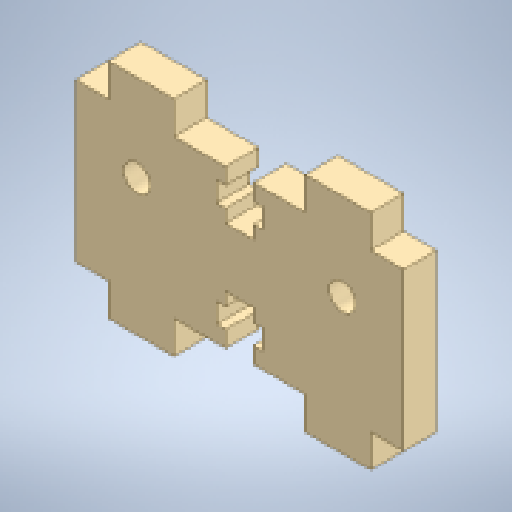
# Autodesk Inventor part: стена_каретки
Saved by Autodesk Inventor 2024 (Build 280153000, 153)
## iProperties
Created: 2026-02-02
Part Number: стена_каретки
Material: Типовые
Document SubType Name: Modeling
Designer: DELL
Density: 1 g/cm^3
Appearance: Пшеничный
Author: DELL
Autodesk Inventor part; units mm, degrees
ref_plane "YZ Plane" through (0, 0, 0) normal (1, 0, 0) x (0, 1, 0)
ref_plane "XZ Plane" through (0, 0, 0) normal (0, 1, 0) x (-1, 0, 0)
ref_plane "XY Plane" through (0, 0, 0) normal (0, 0, 1) x (1, 0, 0)
sketch "Эскиз1" plane through (0, 0, 0) normal (0, 0, 1) x (1, 0, 0)
  line L0 (20, 9.6) -> (-20, 9.6)
  line L1 (-20, 9.6) -> (-20, -9.6)
  line L2 (-20, -9.6) -> (20, -9.6)
  line L3 (20, -9.6) -> (20, 9.6)
  line L4 (20, 9.6) -> (-20, -9.6) construction
  line L5 (-20, 9.6) -> (20, -9.6) construction
  line L6 (-16, 9.6) -> (-8, 9.6)
  line L7 (-8, 9.6) -> (-8, 13.6)
  line L8 (-8, 13.6) -> (-16, 13.6)
  line L9 (-16, 13.6) -> (-16, 9.6)
  line L10 (16, 9.6) -> (8, 9.6)
  line L11 (8, 9.6) -> (8, 13.6)
  line L12 (8, 13.6) -> (16, 13.6)
  line L13 (16, 13.6) -> (16, 9.6)
  line L14 (-16, -9.6) -> (-8, -9.6)
  line L15 (-8, -9.6) -> (-8, -13.6)
  line L16 (-8, -13.6) -> (-16, -13.6)
  line L17 (-16, -13.6) -> (-16, -9.6)
  line L18 (8, -9.6) -> (16, -9.6)
  line L19 (16, -9.6) -> (16, -13.6)
  line L20 (16, -13.6) -> (8, -13.6)
  line L21 (8, -13.6) -> (8, -9.6)
  point P0 (0, 0)
  point P1 (-16, 11.6)
  point P2 (16, -9.6)
  point P3 (8, 9.6)
  point P4 (-8, 9.6)
  dimension "d0" = 40
  dimension "d1" = 19.2
  dimension "d2" = 8
  dimension "d3" = 4
  dimension "d4" = 8
  dimension "d5" = 4
  dimension "d6" = 4
  dimension "d7" = 4
  dimension "d8" = 8
  dimension "d9" = 4
  constraints: 44 end point, 10 parallel, 5 horizontal, 5 perpendicular, 5 point on line, 3 midpoint
  measures "d0" distance of L2.end L1.end
  measures "d1" distance of L1.end L0.end
  measures "d2" distance of L8.end L7.end
  measures "d3" distance of L7.end L6.end
  measures "d4" distance of L11.end L12.end
  measures "d5" distance from line of L1 point (-16, 11.6)
  measures "d6" distance between parallel lines of L13 L3
  measures "d7" distance of L10.end L11.end
  measures "d8" distance of L15.end L16.end
  measures "d9" distance of L14.end L15.end
extrude "Выдавливание1" add sketch "Эскиз1" along normal blind 4
sketch "Эскиз2" plane through (0, 0, 4) normal (0, 0, 1) x (1, 0, 0)
  line L0 (8, 9.6) -> (-8, 9.6) projected
  line L1 (-1.7, 9.6) -> (1.7, 9.6)
  line L2 (1.7, 9.6) -> (1.7, 3.6)
  line L3 (1.7, 3.6) -> (-1.7, 3.6)
  line L4 (-1.7, 3.6) -> (-1.7, 9.6)
  line L5 (0, 9.6) -> (0, 3.6) construction
  line L6 (-2.8, 5.2) -> (2.8, 5.2)
  line L7 (2.8, 5.2) -> (2.8, 7.6)
  line L8 (2.8, 7.6) -> (-2.8, 7.6)
  line L9 (-2.8, 7.6) -> (-2.8, 5.2)
  line L10 (-2.8, 5.2) -> (2.8, 7.6) construction
  line L11 (2.8, 5.2) -> (-2.8, 7.6) construction
  line L12 (-20, 9.6) -> (-20, -9.6) projected
  line L13 (-20, 0) -> (20, 0) construction
  line L14 (20, -9.6) -> (20, 9.6) projected
  line L15 (8, -9.6) -> (-8, -9.6)
  line L16 (-1.7, -9.6) -> (1.7, -9.6)
  line L17 (1.7, -9.6) -> (1.7, -3.6)
  line L18 (1.7, -3.6) -> (-1.7, -3.6)
  line L19 (-1.7, -3.6) -> (-1.7, -9.6)
  line L20 (0, -9.6) -> (0, -3.6) construction
  line L21 (-2.8, -5.2) -> (2.8, -5.2)
  line L22 (2.8, -5.2) -> (2.8, -7.6)
  line L23 (2.8, -7.6) -> (-2.8, -7.6)
  line L24 (-2.8, -7.6) -> (-2.8, -5.2)
  line L25 (-2.8, -5.2) -> (2.8, -7.6) construction
  line L26 (2.8, -5.2) -> (-2.8, -7.6) construction
  point P0 (0, 0)
  point P1 (0, 6.4)
  point P2 (0, -6.4)
  point P3 (1.7, 5.2)
  point P4 (1.7, 7.6)
  point P5 (1.7, 9.6)
  point P6 (-1.7, 7.6)
  point P7 (-1.7, 5.2)
  point P8 (-1.7, -7.6)
  point P9 (1.7, -7.6)
  point P10 (1.7, -5.2)
  point P11 (-1.7, -5.2)
  dimension "d12" = 3.4
  dimension "d13" = 6
  dimension "d14" = 5.6
  dimension "d15" = 2.4
  dimension "d16" = 2
  constraints: 48 end point, 13 symmetric about line, 7 midpoint, 4 parallel, 4 point on line, 2 horizontal, 2 perpendicular
  measures "d12" distance of L2.end L3.end
  measures "d13" distance of L1.end L2.end
  measures "d14" distance of L8.end L7.end
  measures "d15" distance of L7.end L6.end
  measures "d16" distance between parallel lines of L8 L0
extrude "Выдавливание2" cut sketch "Эскиз2" against normal blind 10
sketch "Эскиз3" plane through (0, 0, 0) normal (0, 0, -1) x (-1, 0, 0)
  circle A0 centre (12.5, 3) radius 1.6 projected
  circle A1 centre (-12.5, 3) radius 1.6 projected
  point P0 (0, 0)
extrude "Выдавливание3" cut sketch "Эскиз3" against normal blind 10
